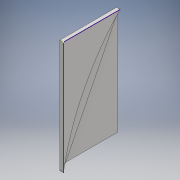
# Autodesk Inventor part: ramps
Saved by Autodesk Inventor 2018 (Build 220112000, 112)
## iProperties
Created: 2019-07-12
Part Number: ramps
Material: Generic
Document SubType Name: Modeling
Designer: Aditya Kendre
Density: 1 g/cm^3
Appearance: Default
Author: Aditya Kendre
Autodesk Inventor part; units mm, degrees
ref_plane "YZ Plane" through (0, 0, 0) normal (1, 0, 0) x (0, 1, 0)
ref_plane "XZ Plane" through (0, 0, 0) normal (0, 1, 0) x (-1, 0, 0)
ref_plane "XY Plane" through (0, 0, 0) normal (0, 0, 1) x (1, 0, 0)
sketch "Sketch1" plane through (0, 0, 0) normal (1, 0, 0) x (0, 1, 0)
  line L0 (0, 0) -> (500, 0)
  line L1 (500, 0) -> (500, -10)
  line L2 (500, -10) -> (0, -10)
  line L3 (0, -10) -> (0, 0)
  line L4 (0, 0) -> (10, 0)
  line L5 (10, 0) -> (10, -1000)
  line L6 (10, -1000) -> (0, -1000)
  line L7 (0, -1000) -> (0, 0)
  arc A0 (500, 0) -> (0, -1000) centre (1931.4141, -1340.707) ccw
  dimension "d0" = 500
  dimension "d1" = 10
  dimension "d2" = 10
  dimension "d3" = 1000
  constraints: 16 end point, 4 parallel, 2 horizontal, 2 perpendicular, 2 point on circle, 1 centre point
  measures "d0" distance of L1.end L2.end
  measures "d1" distance of L0.end L1.end
  measures "d2" distance of L5.end L6.end
  measures "d3" distance of L4.end L5.end
extrude "Extrusion1" add sketch "Sketch1" along normal blind 10 contours L0 L5 L2 L3 | L0 A0 L2 L5 | L2 L5 A0 L7 | L2 A0 L5
sketch "Sketch2" plane through (10, 0, 0) normal (1, 0, 0) x (0, 0, -1)
  point P0 (0, 0)
sketch "Sketch3" plane through (0, 0, 0) normal (-1, 0, 0) x (0, 0, 1)
  line L0 (0, 0) -> (-1000, 0) projected
  line L1 (0, 0) -> (-1000, 0)
  arc A0 (-1000, 0) -> (0, 500) centre (-1340.707, 1931.4141) ccw projected
  line L2 (0, 500) -> (0, 0) projected
  line L3 (0, 500) -> (0, 0)
  line L4 (0, 500) -> (-1000, 0)
  constraints: 6 end point, 2 collinear
extrude "Extrusion2" add sketch "Sketch3" along normal blind 10
sketch "Sketch4" plane through (10, 0, 0) normal (1, 0, 0) x (0, 0, -1)
  line L0 (0, 500) -> (0, 0) projected
  line L1 (0, 500) -> (0, 0)
  line L2 (0, 0) -> (1000, 0) projected
  line L3 (0, 0) -> (1000, 0)
  constraints: 4 end point, 2 collinear
sketch "Sketch5" plane through (-10, 0, 0) normal (-1, 0, 0) x (0, 0, 1)
  line L0 (0, 0) -> (-1000, 0) construction
  line L1 (-1000, 0) -> (-950, 0) construction
  line L2 (-950, 0) -> (-950, 50) construction
  line L3 (-950, 50) -> (-1000, 50) construction
  line L4 (-1000, 50) -> (-1000, 0) construction
  arc A0 (-1000, 0) -> (-950, 50) centre (-1000.9904, 50.9904) ccw
  line L5 (-1000, 0) -> (-950, 0)
  line L6 (-950, 50) -> (-950, 0)
  dimension "d8" = 50
  dimension "d9" = 50
  dimension "d10" = 51
  constraints: 12 end point, 2 collinear, 2 parallel, 2 point on circle, 1 centre point, 1 horizontal, 1 perpendicular
  measures "d8" distance of L3.end L2.end
  measures "d9" distance of L2.end L1.end
  measures "d10" radius of A0
extrude "Extrusion3" add sketch "Sketch5" along normal blind 10
sketch "Sketch6" plane through (-10, 0, 0) normal (-1, 0, 0) x (0, 0, 1)
  line L0 (-950, 0) -> (0, 0) projected
  line L1 (0, 500) -> (0, 0) projected
  line L2 (-950, 0) -> (0, 0)
  line L3 (0, 0) -> (0, 500)
  line L4 (0, 500) -> (-950, 500)
  line L5 (-950, 500) -> (-950, 0)
  constraints: 8 end point, 2 parallel, 1 horizontal, 1 perpendicular
extrude "Extrusion4" add sketch "Sketch6" along normal blind 10
body "Solid1"
